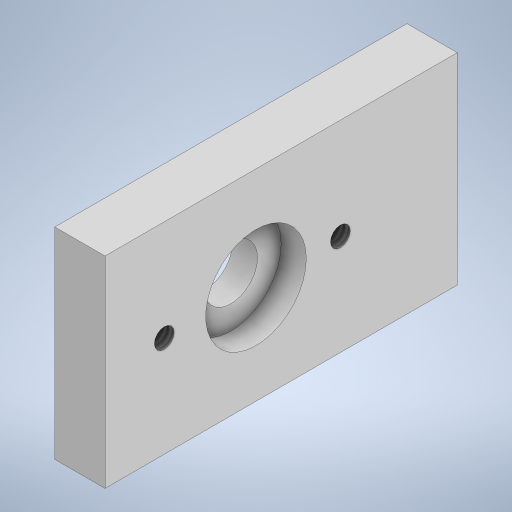
# Autodesk Inventor part: Zero Dead Space Electronic needle valve holder Newst
Saved by Autodesk Inventor 2023 (Build 270158000, 158)
## iProperties
Created: 2022-08-05
Part Number: Zero Dead Space Electronic needle valve holder Newst
Material: Generic
Document SubType Name: Modeling
Designer: dewanlab
Density: 1 g/cm^3
Appearance: Default
Author: dewanlab
Autodesk Inventor part; units mm, degrees
ref_plane "YZ Plane" through (0, 0, 0) normal (1, 0, 0) x (0, 1, 0)
ref_plane "XZ Plane" through (0, 0, 0) normal (0, 1, 0) x (-1, 0, 0)
ref_plane "XY Plane" through (0, 0, 0) normal (0, 0, 1) x (1, 0, 0)
sketch "Sketch1" plane through (0, 0, 0) normal (0, 1, 0) x (-1, 0, 0)
  line L0 (3.1454, 6.687) -> (-3.2046, 6.687)
  line L1 (-3.2046, 6.687) -> (-3.2046, -37.763)
  line L2 (-3.2046, -37.763) -> (3.1454, -37.763)
  line L3 (3.1454, -37.763) -> (3.1454, 6.687)
  point P0 (0, 0)
  dimension "d0" = 6.35
  dimension "d1" = 44.45
  constraints: 8 end point, 2 parallel, 1 horizontal, 1 perpendicular
  measures "d0" distance of L0.start L0.end
  measures "d1" distance of L2.end L0.start
extrude "Extrusion1" add sketch "Sketch1" along normal blind 25.4
sketch "Sketch2" plane through (3.2046, 0, 6.687) normal (1, 0, 0) x (0, 0, -1)
  line L0 (0, 0) -> (0, 25.4) projected
  point P0 (6.687, 0)
  point P1 (19.05, 12.4335)
  dimension "d4" = 19.05
  measures "d4" distance from line of L0 point (19.05, 12.433)
hole "Hole1" at (3.2046, 12.4335, -12.363) direction (-1, 0, 0) diameter 6.7564 end through all counterbore diameter 12.7 counterbore depth 3.175 clearance for "Hex Head Bolt" size "1/4" standard "Ansi Unified Screw Threads"
sketch "Sketch4" plane through (-3.1454, 0, -37.763) normal (-1, 0, 0) x (0, 0, 1)
  line L0 (44.45, 0) -> (44.45, 25.4) projected
  point P0 (37.763, 0)
  point P1 (14.7574, 12.7)
  dimension "d20" = 29.6926
  measures "d20" distance from line of L0 point (14.757, 12.7)
hole "Hole3" at (-3.1454, 12.7, -23.0056) direction (1, 0, 0) diameter 2.4867 end through all thread size "5-40 UNC" class "2B" standard "ANSI Unified Screw Threads"
sketch "Sketch5" plane through (-3.1454, 0, -37.763) normal (-1, 0, 0) x (0, 0, 1)
  line L0 (44.45, 0) -> (44.45, 25.4) projected
  line L1 (0, 25.4) -> (44.45, 25.4) projected
  point P0 (37.763, 0)
  point P1 (36.9824, 12.7)
  dimension "d28" = 7.4676
  dimension "d36" = 12.7
  measures "d28" distance from line of L0 point (36.982, 12.7)
  measures "d36" distance from line of L1 point (36.982, 12.7)
hole "Hole4" at (-3.1454, 12.7, -0.7806) direction (1, 0, 0) diameter 2.4867 end through all thread size "5-40 UNC" class "2B" standard "ANSI Unified Screw Threads"
equation "\"d22\" = d20"
equation "\"d30\" = d28"
body "Solid1"
